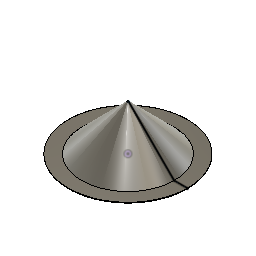
SMB electrode receptacle v29 (Autodesk Fusion 360 archive; units mm, degrees)
design "electrode v2"
Autodesk Fusion 360 part; units mm, degrees
sketch "Sketch1" plane through (0, 0, 0) normal (0, 0, 1) x (1, 0, 0)
  line L0 (0.0652, 3.4348) -> (3.5, 0)
  line L1 (3.5, 0) -> (4.5, 0)
  line L2 (0.0298, 3.3994) -> (3.4793, -0.05)
  line L3 (3.4793, -0.05) -> (4.5, -0.05)
  line L4 (0.0652, 3.4348) -> (0.0298, 3.3994)
  line L5 (4.5, -0.05) -> (4.5, 0)
  dimension "d1" = 3.5
  dimension "d2" = 1
  dimension "d3" = 45
  dimension "d4" = 0.05
  constraint horizontal L1
  constraint horizontal origin L0.end
  constraint perpendicular L1 L5
  measures "d1" distance of origin L0.end
  measures "d2" distance of L0.end L1.end
  measures "d3" angle of L0 L1
revolve "Revolve1" add sketch "Sketch1" angle 360 about axis through (0, 1.75, 0) along (0, 1, 0)

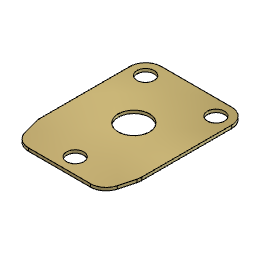
design "smb electrode top ground"
Autodesk Fusion 360 part; units mm, degrees
sketch "Sketch1" plane through (0, 0, 0) normal (0, 1, 0) x (1, 0, 0)
  circle A0 centre (-4.5, 13.5) radius 1.1
  circle A1 centre (4.5, 13.5) radius 1.1
  line L0 (0, -20) -> (0, -2.5) construction
  circle A2 centre (0, 0) radius 1.1
  circle A3 centre (0, 7.5) radius 2
  line L1 (-6.5, -2) -> (6.5, -2)
  line L2 (6.5, -2) -> (6.5, 15.5)
  line L3 (-6.5, -2) -> (-6.5, 15.5)
  line L4 (6.5, 15.5) -> (-6.5, 15.5)
  line L5 (-5.5, -2) -> (-6.5, 1.7321)
  line L6 (5.5, -2) -> (6.5, 1.7321)
  dimension "d1" = 2.2
  dimension "d2" = 2.2
  dimension "d3" = 9
  dimension "d4" = 13.5
  dimension "d5" = 2.2
  dimension "d6" = 7.5
  dimension "d7" = 4
  dimension "d8" = 13
  dimension "d9" = 2
  dimension "d10" = 2
  dimension "d15" = 30
  dimension "d16" = 11
  constraint horizontal A0.centre A1.centre
  constraint symmetric A0.centre A1.centre L0
  constraint coincident A2.centre origin
  constraint vertical A2.centre A3.centre
  constraint horizontal L1
  constraint perpendicular L1 L2
  constraint perpendicular L1 L3
  constraint perpendicular L2 L4
  constraint coincident L1 L5.start
  constraint coincident L3 L5.end
  constraint coincident L1 L6.start
  constraint coincident L2 L6.end
  constraint symmetric L0 L5 L6
  measures "d1" diameter of A0
  measures "d2" diameter of A1
  measures "d3" horizontal distance of A0.centre A1.centre
  measures "d4" vertical distance of A2.centre A1.centre
  measures "d5" diameter of A2
  measures "d6" distance of A2.centre A3.centre
  measures "d7" diameter of A3
  measures "d8" distance of L1.start L1.end
  measures "d9" distance of A2.centre L1
  measures "d10" distance of A1.centre L4
  measures "d15" angle of L5 L6
  measures "d16" distance of L5.start L6.start
extrude "Extrude1" add sketch "Sketch1" along normal blind 0.38 contours L1 L2 L3 L4 L5 L6
fillet "Fillet1" radius 2 6 edges at (-6.5, 0.19, -15.5) (6.5, 0.19, -15.5) (-5.5, 0.19, 2) (-6.5, 0.19, -1.7321) (5.5, 0.19, 2) (6.5, 0.19, -1.7321)

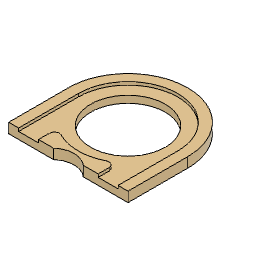
design "smb electrode insulators"
Autodesk Fusion 360 part; units mm, degrees
sketch "Sketch1" plane through (0, 0, 0) normal (0, 1, 0) x (1, 0, 0)
  line L0 (0, 0) -> (12, 0)
  line L1 (12, 0) -> (12, -12)
  line L2 (12, -12) -> (0, -12)
  line L3 (0, -12) -> (0, 0)
  circle A0 centre (6, -6) radius 3.75
  line L4 (6, 0) -> (6, -12) construction
  circle A1 centre (6, -6) radius 5
  line L5 (2, -12) -> (2, -9) construction
  line L6 (1, -12) -> (1, -6)
  line L7 (3, -10) -> (3, -12)
  arc A2 (7.5, -12) -> (4.5, -12) centre (6, -13.7) ccw
  dimension "d1" = 12
  dimension "d2" = 12
  dimension "d3" = 7.5
  dimension "d4" = 10
  dimension "d5" = 4
  dimension "d6" = 2
  dimension "d16" = 3
  dimension "d17" = 1.7
  constraint horizontal L0
  constraint vertical L1
  constraint horizontal L2
  constraint vertical L3
  constraint coincident L0.start L3.end
  constraint midpoint L0 L4.start
  constraint midpoint L2 L4.end
  constraint midpoint A0.centre L4
  constraint concentric A0 A1
  constraint coincident L2 L5.start
  constraint perpendicular L2 L5
  constraint coincident L2 L6.start
  constraint coincident A1 L6.end
  constraint perpendicular L2 L6
  constraint coincident A1 L7.start
  constraint coincident L2 L7.end
  constraint perpendicular L2 L7
  constraint coincident A1 L5.end
  constraint coincident L2 A2.start
  constraint coincident L2 A2.end
  constraint coincident L4 A2.centre
  measures "d1" distance of L0.start L2.end
  measures "d2" distance of L1.end L2.end
  measures "d3" diameter of A0
  measures "d4" diameter of A1
  measures "d5" distance of L4.end L5
  measures "d6" distance of L6 L7
  measures "d16" distance of A2.end A2.start
  measures "d17" distance of L2 A2.centre
extrude "Extrude1" add sketch "Sketch1" against normal blind 1 contours L0 L1 L2 L3 A1 L6 L7 A2 | L2 A1 L6 L7 | A1
extrude "Extrude2" cut sketch "Sketch1" against normal blind 0.3 contours A1
extrude "Extrude3" cut sketch "Sketch1" against normal blind 0.3 contours L2 A1 L6 L7
ref_plane "WorkPlane1" through (6, -0.5, 6) normal (1, 0, 0) x (0, 0, 1)
mirror "Mirror1" about plane through (6, -0.5, 6) normal (1, 0, 0) of "Extrude3"
fillet "Fillet1" radius 6 2 edges at (0, -0.5, 0) (12, -0.5, 0)
fillet "Fillet2" radius 0.5 2 edges at (3, -0.15, 10) (9, -0.15, 10)
equation "d3 = ( 3.75 * 2 ) * 1 mm"

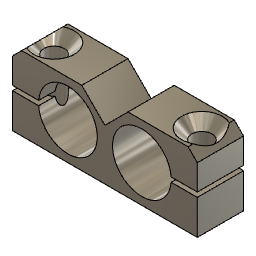
design "SMB plug holder"
Autodesk Fusion 360 part; units mm, degrees
sketch "Sketch1" plane through (0, 0, 0) normal (0, 0, 1) x (1, 0, 0)
  line L0 (0, 0) -> (20, 0)
  line L1 (20, 0) -> (20, 8)
  line L2 (20, 8) -> (0, 8)
  line L3 (0, 8) -> (0, 0)
  circle A0 centre (6, 4) radius 3.175
  circle A1 centre (14, 4) radius 3.175
  line L4 (10, 0) -> (10, 8) construction
  line L5 (7.5, 8) -> (10, 5.5)
  line L6 (10, 5.5) -> (12.5, 8)
  dimension "d1" = 6.35
  dimension "d2" = 6.35
  dimension "d3" = 8
  dimension "d4" = 4
  dimension "d5" = 20
  dimension "d6" = 8
  dimension "d9" = 2.5
  constraint horizontal L0
  constraint vertical L1
  constraint horizontal L2
  constraint vertical L3
  constraint coincident L0.start L3.end
  constraint horizontal A0.centre A1.centre
  constraint midpoint L0 L4.start
  constraint midpoint L2 L4.end
  constraint symmetric A0.centre A1.centre L4
  constraint coincident L2 L5.start
  constraint coincident L4 L5.end
  constraint coincident L2 L6.end
  constraint perpendicular L5 L6
  constraint symmetric L4 L5 L6
  measures "d1" diameter of A0
  measures "d2" diameter of A1
  measures "d3" distance of A0.centre A1.centre
  measures "d4" distance of L0 A0.centre
  measures "d5" distance of L0.start L0.end
  measures "d6" distance of L0 L2
  measures "d9" distance of L2 L5.end
extrude "Extrude1" add sketch "Sketch1" against normal blind 5 contours L0 L1 L2 L3 L5 L6
sketch "Sketch2" plane through (0, 8, 0) normal (0, 1, 0) x (-1, 0, 0)
  line L0 (-12.5, 0) -> (-20, 0)
  line L1 (-20, 0) -> (-20, -5)
  line L2 (-20, -5) -> (-12.5, -5)
  line L3 (-12.5, -5) -> (-12.5, 0)
  line L4 (0, 0) -> (0, -5)
  line L5 (-20, 0) -> (-20, -5)
  line L6 (-20, -2.5) -> (0, -2.5) construction
  line L7 (-10, 0) -> (-10, -5)
  point P0 (-2, -2.5)
  point P1 (-18, -2.5)
  dimension "d10" = 2
  dimension "d19" = 16
  constraint midpoint L1 L6.start
  constraint midpoint L4 L6.end
  constraint coincident L6 P0
  constraint coincident L6 P1
  constraint symmetric P0 P1 L7
  measures "d10" distance of L4 P0
  measures "d19" distance of P0 P1
chamfer "Chamfer1" distance 1 angle 45 2 edges at (20, 8, -2.5) (0, 8, -2.5)
hole "Hole1" at (2, 8, -2.5) at (18, 8, -2.5) direction (0, -1, 0) diameter 2.2 depth 10 tip angle 118 countersink diameter 4.4 countersink angle 90
ref_plane "WorkPlane1" through (16.25, 4, -2.5) normal (0, 1, 0) x (1, 0, 0)
sketch "Sketch3" plane through (16.25, 4, -3.5) normal (0, 1, 0) x (1, 0, 0)
  line L0 (0, 6) -> (6.8751, 6)
  line L1 (6.8751, 6) -> (6.8751, -6.5674)
  line L2 (6.8751, -6.5674) -> (0, -6.5674)
  line L3 (0, -6.5674) -> (0, 6)
  line L4 (-17, 6) -> (-11.0861, 6)
  line L5 (-11.0861, 6) -> (-11.0861, -6.5674)
  line L6 (-11.0861, -6.5674) -> (-17, -6.5674)
  line L7 (-17, -6.5674) -> (-17, 6)
  constraint horizontal L0
  constraint vertical L1
  constraint horizontal L2
  constraint vertical L3
  constraint horizontal L4
  constraint vertical L5
  constraint horizontal L6
  constraint vertical L7
extrude "Extrude2" cut sketch "Sketch3" along normal mid plane 0.5
